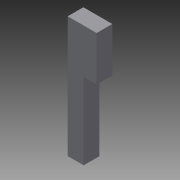
# Autodesk Inventor part: Linear Actuator
Saved by Autodesk Inventor 2015 (Build 190159000, 159)
## iProperties
Created: 2015-01-31
Part Number: Linear Actuator
Material: Generic
Document SubType Name: Modeling
Designer: chapale16
Density: 1 g/cm^3
Appearance: Default
Author: chapale16
Autodesk Inventor part; units mm, degrees
ref_plane "YZ Plane" through (0, 0, 0) normal (1, 0, 0) x (0, 1, 0)
ref_plane "XZ Plane" through (0, 0, 0) normal (0, 1, 0) x (-1, 0, 0)
ref_plane "XY Plane" through (0, 0, 0) normal (0, 0, 1) x (1, 0, 0)
sketch "Sketch1" plane through (0, 0, 0) normal (0, 0, 1) x (1, 0, 0)
  line L0 (0, 0) -> (73.66, 0)
  line L1 (73.66, 0) -> (73.66, -308.102)
  line L2 (73.66, -308.102) -> (0, -308.102)
  line L3 (0, -308.102) -> (0, 0)
  dimension "d0" = 73.66
  dimension "d1" = 308.102
  constraints: 8 end point, 2 perpendicular, 1 horizontal, 1 vertical
  measures "d0" distance of L0.start L0.end
  measures "d1" distance of L0.end L1.end
extrude "Extrusion1" add sketch "Sketch1" along normal blind 39.878
sketch "Sketch2" plane through (0, 0, 39.878) normal (0, 0, 1) x (1, 0, 0)
  line L0 (73.66, 0) -> (73.66, -96.266)
  line L1 (73.66, -308.102) -> (73.66, 0) projected
  line L2 (73.66, -96.266) -> (73.66, -308.102)
  line L3 (73.66, -308.102) -> (40.64, -308.102)
  line L4 (0, -308.102) -> (73.66, -308.102) projected
  line L5 (73.66, -113.4326) -> (40.64, -113.4326)
  line L6 (40.64, -113.4326) -> (40.64, -308.102)
  point P0 (0, 0)
  dimension "d4" = 96.266
  dimension "d5" = 33.02
  dimension "d6" = 33.02
  constraints: 10 end point, 3 point on line, 1 collinear, 1 perpendicular
  measures "d4" distance of L0.start L0.end
  measures "d5" distance of L1.start L3.end
  measures "d6" distance of L5.start L5.end
extrude "Extrusion2" cut sketch "Sketch2" against normal through all
body "Solid1"
